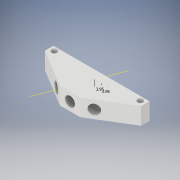
# Autodesk Inventor part: Subbase
Saved by Autodesk Inventor 2018 (Build 220112000, 112)
## iProperties
Created: 2018-01-25
Part Number: Subbase
Material: PAEK Plastic
Document SubType Name: Modeling
Designer: ERSKINA
Density: 1.32 g/cm^3
Appearance: Smooth - White
Author: ERSKINA
Autodesk Inventor part; units mm, degrees
ref_plane "YZ Plane" through (0, 0, 0) normal (1, 0, 0) x (0, 1, 0)
ref_plane "XZ Plane" through (0, 0, 0) normal (0, 1, 0) x (-1, 0, 0)
ref_plane "XY Plane" through (0, 0, 0) normal (0, 0, 1) x (1, 0, 0)
sketch "Sketch1" plane through (0, 0, 0) normal (0, 1, 0) x (-1, 0, 0)
  line L0 (0, 0) -> (28.25, 0)
  line L1 (28.25, 0) -> (28.25, 5)
  line L2 (28.25, 5) -> (6, 18.5)
  line L3 (6, 18.5) -> (0, 18.5)
  line L4 (0, 18.5) -> (-6, 18.5)
  line L5 (-6, 18.5) -> (-28.25, 5)
  line L6 (-28.25, 5) -> (-28.25, 0)
  line L7 (-28.25, 0) -> (0, 0)
  dimension "d0" = 28.25
  dimension "d1" = 28.25
  dimension "d2" = 18.5
  dimension "d3" = 6
  dimension "d4" = 6
  dimension "d5" = 5
  constraints: 16 end point, 2 horizontal, 2 parallel, 1 collinear, 1 perpendicular
  measures "d0" distance of L0.start L0.end
  measures "d1" distance of L0.start L6.end
  measures "d2" distance of L0.start L3.end
  measures "d3" distance of L4.end L3.end
  measures "d4" distance of L2.end L3.end
  measures "d5" distance of L1.end L0.end
extrude "Extrusion1" add sketch "Sketch1" along normal blind 10
sketch "Sketch2" plane through (0, 10, 0) normal (0, 1, 0) x (1, 0, 0)
  circle A0 centre (-25.25, -2.5) radius 1.6
  line L0 (-28.25, 0) -> (-28.25, -5) projected
  line L1 (28.25, 0) -> (-28.25, 0) projected
  circle A1 centre (25.25, -2.5) radius 1.6
  line L2 (28.25, -5) -> (28.25, 0) projected
  point P0 (0, 0)
  dimension "d8" = 3.2
  dimension "d9" = 3
  dimension "d10" = 2.5
  dimension "d11" = 3.2
  dimension "d12" = 3
  constraints: 2 centre point
  measures "d8" diameter of A0
  measures "d9" distance from line of L0 A0.centre
  measures "d10" distance from line of L1 A0.centre
  measures "d11" diameter of A1
  measures "d12" distance from line of A1.centre L2
extrude "Extrusion2" cut sketch "Sketch2" against normal blind 10
sketch "Sketch3" plane through (-6, 0, 18.5) normal (0, 0, 1) x (1, 0, 0)
  circle A0 centre (6, 5) radius 2.8804
  line L0 (0, 10) -> (12, 10) projected
  point P0 (6, 0)
  dimension "d15" = 5.7607
  dimension "d16" = 5
  constraints: 1 centre point
  measures "d15" diameter of A0
  measures "d16" distance from line of L0 A0.centre
extrude "Extrusion3" cut sketch "Sketch3" against normal blind 7
thread "Thread1" size "1/4-28 UNF" class "2B" standard "ANSI Unified Screw Threads" full length
sketch "Sketch4" plane through (-6, 0, 18.5) normal (-0.5187274, 0, 0.8549397) x (0.8549397, 0, 0.5187274)
  circle A0 centre (-6, 5) radius 2.8805
  line L0 (0, 0) -> (0, 10) projected
  line L1 (-26.0252, 10) -> (0, 10) projected
  point P0 (-4.4668, 0)
  dimension "d21" = 5.761
  dimension "d22" = 6
  dimension "d23" = 5
  constraints: 1 centre point
  measures "d21" diameter of A0
  measures "d22" distance from line of L0 A0.centre
  measures "d23" distance from line of L1 A0.centre
extrude "Extrusion4" cut sketch "Sketch4" against normal blind 7
sketch "Sketch5" plane through (28.25, 0, 5) normal (0.5187274, 0, 0.8549397) x (0.8549397, 0, -0.5187274)
  circle A0 centre (-20.0252, 5) radius 2.8805
  line L0 (-26.0252, 10) -> (0, 10) projected
  line L1 (-26.0252, 0) -> (-26.0252, 10) projected
  point P0 (-21.5584, 0)
  dimension "d26" = 5.761
  dimension "d27" = 5
  dimension "d28" = 6
  constraints: 1 centre point
  measures "d26" diameter of A0
  measures "d27" distance from line of L0 A0.centre
  measures "d28" distance from line of L1 A0.centre
extrude "Extrusion5" cut sketch "Sketch5" against normal blind 7
thread "Thread2" size "1/4-28 UNF" class "2B" standard "ANSI Unified Screw Threads" full length
thread "Thread3" size "1/4-28 UNF" class "2B" standard "ANSI Unified Screw Threads" full length
sketch "Sketch6" plane through (0, 5, 11.5) normal (0, 0, 1) x (1, 0, 0)
  circle A0 centre (0, 0) radius 0.75
  point P0 (0, -5)
  dimension "d35" = 1.5
  constraints: 1 centre point
  measures "d35" diameter of A0
extrude "Extrusion6" cut sketch "Sketch6" against normal blind 12
sketch "Sketch14" plane through (-7.4985, 5, 9.4031) normal (-0.5187274, 0, 0.8549397) x (0.8549397, 0, 0.5187274)
  point P0 (1.5332, -5)
  point P1 (0, 0)
sketch "Sketch19" plane through (28.25, 0, 0) normal (0, 0, -1) x (-1, 0, 0)
  circle A0 centre (28.25, 5) radius 0.75 projected
  point P0 (28.25, 0)
  point P1 (32.2, 5)
  dimension "d50" = 3.95
  measures "d50" distance of A0.centre point (32.2, 5)
sketch3d "3D Sketch5"
hole "Hole1" at (-7.4985, 5, 9.4031) direction (0.3530766, 0, -0.9355944) diameter 1.778 depth 20.2512 tip angle 110 start extended yes
sketch "Sketch20" plane through (28.25, 0, 0) normal (0, 0, -1) x (-1, 0, 0)
  circle A0 centre (28.25, 5) radius 0.75 projected
  point P0 (28.25, 0)
  point P1 (24.3, 5)
  dimension "d62" = 3.95
  measures "d62" distance of A0.centre point (24.3, 5)
sketch "Sketch21" plane through (7.4985, 5, 9.4031) normal (0.5187274, 0, 0.8549397) x (0.8549397, 0, -0.5187274)
  point P0 (-1.5332, -5)
  point P1 (0, 0)
sketch3d "3D Sketch6"
hole "Hole2" at (7.4985, 5, 9.4031) direction (-0.3530766, 0, -0.9355944) diameter 1.5 depth 20.2512 tip angle 110 start extended yes
sketch "Sketch23" plane through (28.25, 0, 0) normal (0, 0, -1) x (-1, 0, 0)
  circle A0 centre (11.25, 5) radius 1.25
  circle A1 centre (28.25, 5) radius 0.75 projected
  circle A2 centre (40.75, 5) radius 1.25
  point P0 (28.25, 0)
  dimension "d72" = 2.5
  dimension "d73" = 17
  dimension "d74" = 2.5
  dimension "d75" = 12.5
  constraints: 2 centre point
  measures "d72" diameter of A0
  measures "d73" distance of A1.centre A0.centre
  measures "d74" diameter of A2
  measures "d75" distance of A2.centre A1.centre
extrude "Extrusion7" cut sketch "Sketch23" against normal blind 5 contours A0 | A2
thread "Thread4" size "M3x0.5" class "6H" standard "ANSI Metric M Profile" full length
thread "Thread5" size "M3x0.5" class "6H" standard "ANSI Metric M Profile" full length
body "Solid1"
